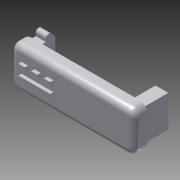
# Autodesk Inventor part: rubber-flippity-flap
Saved by Autodesk Inventor 2015 (Build 190159000, 159)
## iProperties
Created: 2014-12-10
Part Number: rubber-flippity-flap
Material: Nylon 6/6
Document SubType Name: Modeling
Designer: Adam
Density: 1.13 g/cm^3
Appearance: White
Author: Adam
Autodesk Inventor part; units mm, degrees
ref_plane "YZ Plane" through (0, 0, 0) normal (1, 0, 0) x (0, 1, 0)
ref_plane "XZ Plane" through (0, 0, 0) normal (0, 1, 0) x (-1, 0, 0)
ref_plane "XY Plane" through (0, 0, 0) normal (0, 0, 1) x (1, 0, 0)
sketch "Sketch1" plane through (0, 0, 0) normal (0, 0, 1) x (1, 0, 0)
  line L0 (10, 0) -> (10, 2) projected
  arc A0 (10, 2) -> (8.5, 3.5) centre (8.5, 2) ccw projected
  line L1 (8.5, 3.5) -> (-8.5, 3.5) projected
  arc A1 (-8.5, 3.5) -> (-10, 2) centre (-8.5, 2) ccw projected
  line L2 (-10, 2) -> (-8, 2) projected
  line L3 (-8, 2) -> (-8, 0) projected
  line L4 (-6, 0) -> (-8, 0) projected
  arc A2 (0, 0) -> (-6, 0) centre (-3, 0) ccw projected
  line L5 (7, 0) -> (0, 0) projected
  line L6 (7, 0) -> (7, 2.5) projected
  line L7 (7, 2.5) -> (9, 2.5) projected
  line L8 (9, 2.5) -> (9, 0) projected
  line L9 (10, 0) -> (9, 0) projected
  line L10 (-8, -2) -> (-10, -2) projected
  arc A3 (-10, -2) -> (-8.5, -3.5) centre (-8.5, -2) ccw projected
  line L11 (8.5, -3.5) -> (-8.5, -3.5) projected
  arc A4 (8.5, -3.5) -> (10, -2) centre (8.5, -2) ccw projected
  line L12 (10, 0) -> (10, -2) projected
  line L13 (9, 0) -> (10, 0) projected
  line L14 (9, 0) -> (9, -2.5) projected
  line L15 (9, -2.5) -> (7, -2.5) projected
  line L16 (7, -2.5) -> (7, 0) projected
  line L17 (0, 0) -> (7, 0) projected
  arc A5 (-6, 0) -> (0, 0) centre (-3, 0) ccw projected
  line L18 (-8, 0) -> (-6, 0) projected
  line L19 (-8, 0) -> (-8, -2) projected
  line L20 (-10, 2) -> (-10, 0) projected
  line L21 (-10, -2) -> (-10, 0) projected
  circle A6 centre (-8.5, 2) radius 1.25
  circle A7 centre (-8.5, -2) radius 1.25
  circle A8 centre (8.5, -2) radius 1.25
  circle A9 centre (8.5, 2) radius 1.25
  line L22 (8.5, 3.25) -> (-8.5, 3.25)
  line L23 (-9.75, 2) -> (-9.75, -2)
  line L24 (-8.5, -3.25) -> (8.5, -3.25)
  line L25 (9.75, 2) -> (9.75, -2)
  dimension "d22" = 0.25
  constraints: 8 end point, 8 point on circle, 7 tangent, 4 centre point, 4 coincident, 2 parallel, 2 point on line
  measures "d22" radial gap between concentric circles of A0 A9
extrude "Extrusion1" add sketch "Sketch1" along normal blind 2 contours L25 A8 L14 L9 | L9 L8 A9 L25 | L14 A8 L15 L16 L6 L7 A9 L8 | A9 L8 L7 | A8 L15 L14 | A9 L7 L8 | L14 L15 A8 | A9 L7 L6 L5 A2 L4 L3 A6 L22 | L24 A7 L19 L4 A5 L5 L16 L15 A8 | A6 L3 L2 | A7 L10 L19 | L2 L3 A6 | A6 L3 L19 A7 L23 | A7 L19 L10 | A5 A2
sketch "Sketch2" plane through (0, 0, 0) normal (0, 0, -1) x (-1, 0, 0)
  line L0 (-9, -2.5) -> (-7, -2.5) projected
  line L1 (-9, 2.5) -> (-9, 0) projected
  line L2 (-7, 2.5) -> (-9, 2.5) projected
  line L3 (-7, 0) -> (-7, 2.5) projected
  line L4 (-7, -2.5) -> (-7, 0) projected
  line L5 (-9, 0) -> (-9, -2.5) projected
  point P0 (0, 0)
extrude "Extrusion2" add sketch "Sketch2" along normal blind 4
sketch "Sketch3" plane through (0, 0, 0) normal (0, 0, -1) x (-1, 0, 0)
  line L0 (8, 2) -> (8, 0) projected
  line L1 (8, 0) -> (8, -2) projected
  line L2 (8, -2) -> (10, -2) projected
  line L3 (10, -2) -> (10, 0) projected
  line L4 (10, 2) -> (10, 0) projected
  line L5 (10, 2) -> (8, 2) projected
  line L6 (9.8, -1.8) -> (8.2, -1.8)
  line L7 (8.2, -1.8) -> (8.2, 1.8)
  line L8 (8.2, 1.8) -> (9.8, 1.8)
  line L9 (9.8, 1.8) -> (9.8, -1.8)
  point P0 (0, 0)
  dimension "d5" = 0.2
  dimension "d6" = 0.2
  dimension "d7" = 0.2
  dimension "d8" = 0.2
  constraints: 8 end point, 2 parallel, 1 horizontal, 1 perpendicular
  measures "d5" distance between parallel lines of L5 L8
  measures "d6" distance between parallel lines of L2 L6
  measures "d7" distance between parallel lines of L1 L7
  measures "d8" distance between parallel lines of L4 L9
extrude "Extrusion3" add sketch "Sketch3" along normal blind 3.5 contours L6 L7 L8 L9
sketch "Sketch4" plane through (-9.8, -1.8, 0) normal (-1, 0, 0) x (0, 0, 1)
  line L0 (-3.5, 0) -> (-3.5, 3.6) projected
  line L1 (0, 3.6) -> (-3.5, 3.6) projected
  line L2 (0, 0) -> (-3.5, 0) projected
  line L3 (-3.5, 0) -> (-2, -1.2586)
  line L4 (-2, -1.2586) -> (-2, 5.3876)
  line L5 (-2, 5.3876) -> (-3.5, 3.6)
  point P0 (0, 1.8)
  dimension "d11" = 50
  dimension "d12" = 50
  dimension "d13" = 1.5
  constraints: 6 end point, 1 vertical
  measures "d11" angle of L1 L5
  measures "d12" angle of L3 L0
  measures "d13" distance between parallel lines of L0 L4
extrude "Extrusion4" add sketch "Sketch4" against normal up to surface (1.6 mm away)
fillet "Fillet2" radius 1 2 edges at (-9, -1.8, -3.5) (-9, 1.8, -3.5)
fillet "Fillet3" radius 0.5 2 edges at (-9, 3.5876, -2) (-9, -3.0586, -2)
fillet "Fillet4" radius 1 5 edges at (9.3839, 2.8839, 2) (9.75, 0, 2) (9.3839, -2.8839, 2) (0, -3.25, 2) (0, 3.25, 2)
sketch "Sketch7" plane through (0, 0, 2) normal (0, 0, 1) x (1, 0, 0)
  line L0 (-6.9276, 0) -> (0, 0) construction
  line L1 (-8, -1.2) -> (-3, -1.2)
  line L2 (-3, -1.2) -> (-3, -0.4)
  line L3 (-3, -0.4) -> (-8, -0.4)
  line L4 (-8, -0.4) -> (-8, -1.2)
  line L5 (-8, 1.2) -> (-7, 1.2)
  line L6 (-7, 1.2) -> (-7, 0.4)
  line L7 (-7, 0.4) -> (-8, 0.4)
  line L8 (-8, 0.4) -> (-8, 1.2)
  line L9 (-6, 0.4) -> (-6, 1.2)
  line L10 (-4, 1.2) -> (-3, 1.2)
  line L11 (-3, 1.2) -> (-3, 0.4)
  line L12 (-3, 0.4) -> (-4, 0.4)
  line L13 (-4, 0.4) -> (-4, 1.2)
  line L14 (-6, 1.2) -> (-5, 1.2)
  line L15 (-5, 1.2) -> (-5, 0.4)
  line L16 (-5, 0.4) -> (-6, 0.4)
  dimension "d31" = 5
  dimension "d32" = 0.8
  dimension "d33" = 0.4
  dimension "d35" = 0.8
  dimension "d36" = 1
  dimension "d37" = 1
  dimension "d38" = 1
  dimension "d39" = 1
  dimension "d40" = 1
  dimension "d41" = 3
  dimension "d42" = 0.4
  constraints: 34 end point, 6 parallel, 5 horizontal, 5 perpendicular, 3 collinear, 2 point on line
  measures "d31" distance of L1.start L1.end
  measures "d32" distance between parallel lines of L1 L3
  measures "d33" distance between parallel lines of L3 L0
  measures "d35" distance between parallel lines of L7 L5
  measures "d36" distance between parallel lines of L6 L8
  measures "d37" distance between parallel lines of L9 L6
  measures "d38" distance between parallel lines of L9 L15
  measures "d39" distance between parallel lines of L11 L13
  measures "d40" distance between parallel lines of L15 L13
  measures "d41" distance from line of L0.end L2
  measures "d42" distance between parallel lines of L7 L0
extrude "Extrusion6" add sketch "Sketch7" along normal blind 0.5
sketch "Sketch8" plane through (0, 0, 2) normal (0, 0, 1) x (1, 0, 0)
  line L0 (-1, 1.5561) -> (6.4631, 1.5561) construction
  line L1 (6.4631, 1.5561) -> (6.4631, -1.5561) construction
  line L2 (6.4631, -1.5561) -> (-1, -1.5561) construction
  line L3 (-1, -1.5561) -> (-1, 1.5561) construction
  line L4 (1.4132, -1.5512) -> (-0.5999, -1.5512)
  line L5 (-0.5999, -1.5512) -> (-0.5999, -1.0201)
  line L6 (-0.5999, -1.0201) -> (0.0423, -1.0201)
  line L7 (0.0423, -1.0201) -> (0.0423, 0.5928)
  line L8 (0.0423, 0.5928) -> (-0.5999, 0.5928)
  line L9 (-0.5999, 0.5928) -> (-0.5999, 1.0893)
  spline S0 degree 2 poles (-0.5999, 1.0893) (-0.4591, 1.0893) (-0.18, 1.1263) (-0.096, 1.1658) knots 0 0 0 1 2 2 2
  spline S1 degree 2 poles (-0.096, 1.1658) (0.0004, 1.2152) (0.109, 1.3807) (0.1189, 1.5042) knots 0 0 0 1 2 2 2
  line L10 (0.1189, 1.5042) -> (0.7858, 1.5042)
  line L11 (0.7858, 1.5042) -> (0.7858, -1.0201)
  line L12 (0.7858, -1.0201) -> (1.4132, -1.0201)
  line L13 (1.4132, -1.0201) -> (1.4132, -1.5512)
  line L14 (4.2191, -1.5512) -> (1.9788, -1.5512)
  line L15 (1.9788, -1.5512) -> (1.9788, -1.0547)
  spline S2 degree 2 poles (1.9788, -1.0547) (2.2629, -0.8275) (2.7174, -0.4273) (2.8878, -0.247) knots 0 0 0 1 2 2 2
  spline S3 degree 2 poles (2.8878, -0.247) (3.1126, -0.0124) (3.3126, 0.3458) (3.3126, 0.5335) knots 0 0 0 1 2 2 2
  spline S4 degree 2 poles (3.3126, 0.5335) (3.3126, 0.7459) (3.0582, 0.9732) (2.831, 0.9732) knots 0 0 0 1 2 2 2
  spline S5 degree 2 poles (2.831, 0.9732) (2.7149, 0.9732) (2.5074, 0.9164) (2.4012, 0.8719) knots 0 0 0 1 2 2 2
  spline S6 degree 2 poles (2.4012, 0.8719) (2.2975, 0.825) (2.1493, 0.7262) (2.1122, 0.7015) knots 0 0 0 1 2 2 2
  line L16 (2.1122, 0.7015) -> (2.0529, 0.7015)
  line L17 (2.0529, 0.7015) -> (2.0529, 1.3659)
  spline S7 degree 2 poles (2.0529, 1.3659) (2.1814, 1.4277) (2.7297, 1.5561) (2.9841, 1.5561) knots 0 0 0 1 2 2 2
  spline S8 degree 2 poles (2.9841, 1.5561) (3.5275, 1.5561) (4.0858, 1.072) (4.0858, 0.6348) knots 0 0 0 1 2 2 2
  spline S9 degree 2 poles (4.0858, 0.6348) (4.0858, 0.3656) (3.8314, -0.1531) (3.5374, -0.4495) knots 0 0 0 1 2 2 2
  spline S10 degree 2 poles (3.5374, -0.4495) (3.3522, -0.6323) (3.0039, -0.9164) (2.9273, -0.9757) knots 0 0 0 1 2 2 2
  line L18 (2.9273, -0.9757) -> (4.2191, -0.9757)
  line L19 (4.2191, -0.9757) -> (4.2191, -1.5512)
  line L20 (7.2005, 1.4968) -> (6.1532, -1.5512)
  line L21 (6.1532, -1.5512) -> (5.3554, -1.5512)
  line L22 (5.3554, -1.5512) -> (4.3081, 1.4968)
  line L23 (4.3081, 1.4968) -> (5.1009, 1.4968)
  line L24 (5.1009, 1.4968) -> (5.7654, -0.5706)
  line L25 (5.7654, -0.5706) -> (6.4273, 1.4968)
  line L26 (6.4273, 1.4968) -> (7.2005, 1.4968)
  point P0 (0, 0)
  dimension "d45" = 3.1122
  dimension "d46" = 1.5561
  dimension "d47" = 1
  constraints: 2 other
  measures "d45" distance between parallel lines of L2 L0
  measures "d46" distance from line of point (0, 0) L2
  measures "d47" distance from line of point (0, 0) L3
extrude "Extrusion7" add sketch "Sketch8" along normal blind 0.5
equation "\"d6\" = d5"
equation "\"d7\" = d6"
equation "\"d8\" = d5"
equation "\"d12\" = d11"
equation "\"d33\" = 0.5 * d32"
equation "\"d35\" = d32"
equation "\"d36\" = 0.2 * d31"
equation "\"d37\" = d36"
equation "\"d38\" = d36"
equation "\"d39\" = d36"
equation "\"d40\" = d36"
equation "\"d42\" = d33"
equation "\"d46\" = 0.5 * d45"
body "Solid1"
